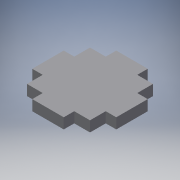
# Autodesk Inventor part: Part4
Saved by Autodesk Inventor 2018 (Build 220112000, 112)
## iProperties
Created: 2018-05-22
Part Number: Part4
Material: Generic
Document SubType Name: Modeling
Designer: Administrator
Density: 1 g/cm^3
Appearance: Default
Author: Administrator
Autodesk Inventor part; units mm, degrees
ref_plane "YZ Plane" through (0, 0, 0) normal (1, 0, 0) x (0, 1, 0)
ref_plane "XZ Plane" through (0, 0, 0) normal (0, 1, 0) x (-1, 0, 0)
ref_plane "XY Plane" through (0, 0, 0) normal (0, 0, 1) x (1, 0, 0)
sketch "Sketch1" plane through (0, 0, 0) normal (0, 1, 0) x (-1, 0, 0)
  line L0 (-87.6102, -27.7315) -> (-106.6602, -27.7315)
  line L1 (-106.6602, -27.7315) -> (-106.6602, -46.7815)
  line L2 (-106.6602, -46.7815) -> (-87.6102, -46.7815)
  line L3 (-87.6102, -46.7815) -> (-87.6102, -27.7315)
  line L4 (-106.6602, -32.494) -> (-109.8352, -32.494)
  line L5 (-109.8352, -32.494) -> (-109.8352, -42.019)
  line L6 (-109.8352, -42.019) -> (-106.6602, -42.019)
  line L7 (-106.6602, -42.019) -> (-106.6602, -32.494)
  line L8 (-101.8977, -46.7815) -> (-92.3727, -46.7815)
  line L9 (-92.3727, -46.7815) -> (-92.3727, -49.9565)
  line L10 (-92.3727, -49.9565) -> (-101.8977, -49.9565)
  line L11 (-101.8977, -49.9565) -> (-101.8977, -46.7815)
  line L12 (-87.6102, -32.494) -> (-84.4352, -32.494)
  line L13 (-84.4352, -32.494) -> (-84.4352, -42.019)
  line L14 (-84.4352, -42.019) -> (-87.6102, -42.019)
  line L15 (-87.6102, -42.019) -> (-87.6102, -32.494)
  line L16 (-101.8977, -27.7315) -> (-92.3727, -27.7315)
  line L17 (-92.3727, -27.7315) -> (-92.3727, -24.5565)
  line L18 (-92.3727, -24.5565) -> (-101.8977, -24.5565)
  line L19 (-101.8977, -24.5565) -> (-101.8977, -27.7315)
  point P0 (0, 0)
  dimension "d0" = 19.05
  dimension "d1" = 19.05
  dimension "d2" = 3.175
  dimension "d3" = 4.7625
  dimension "d4" = 4.7625
  dimension "d5" = 4.7625
  dimension "d6" = 3.175
  dimension "d7" = 4.7625
  dimension "d8" = 3.175
  dimension "d9" = 4.7625
  dimension "d10" = 3.175
  constraints: 40 end point, 10 parallel, 5 horizontal, 5 perpendicular, 4 point on line
  measures "d0" distance between parallel lines of L2 L0
  measures "d1" distance between parallel lines of L1 L3
  measures "d2" distance between parallel lines of L1 L5
  measures "d3" distance between parallel lines of L2 L6
  measures "d4" distance between parallel lines of L0 L4
  measures "d5" distance between parallel lines of L1 L11
  measures "d6" distance between parallel lines of L10 L2
  measures "d7" distance between parallel lines of L9 L3
  measures "d8" distance between parallel lines of L15 L13
  measures "d9" distance between parallel lines of L2 L14
  measures "d10" distance between parallel lines of L16 L18
extrude "Extrusion1" add sketch "Sketch1" along normal blind 3.175
body "Solid1"
